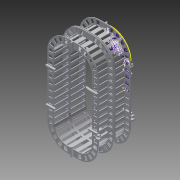
# Autodesk Inventor part: coil_former_hv_new
Saved by Autodesk Inventor 2014 SP1 (Build 180222100, 222)
## iProperties
Created: 2016-09-07
Part Number: coil_former_hv_new
Material: ABS Plastic
Document SubType Name: Modeling
Designer: tguillod
Density: 1.06 g/cm^3
Appearance: Smooth - White
Author: tguillod
Autodesk Inventor part; units mm, degrees
ref_plane "YZ Plane" through (0, 0, 0) normal (1, 0, 0) x (0, 1, 0)
ref_plane "XZ Plane" through (0, 0, 0) normal (0, 1, 0) x (-1, 0, 0)
ref_plane "XY Plane" through (0, 0, 0) normal (0, 0, 1) x (1, 0, 0)
sketch "Sketch1" plane through (0, 0, 0) normal (0, 0, 1) x (1, 0, 0)
  line L0 (0, 0) -> (10, 0)
  line L1 (10, 0) -> (10, 1)
  line L2 (10, 1) -> (1, 1)
  line L3 (1, 1) -> (1, 24.25)
  line L4 (1, 24.25) -> (10, 24.25)
  line L5 (10, 24.25) -> (10, 25.25)
  line L6 (10, 25.25) -> (1, 25.25)
  line L7 (1, 25.25) -> (1, 26.25)
  line L8 (1, 26.25) -> (10, 26.25)
  line L9 (10, 26.25) -> (10, 27.25)
  line L10 (10, 27.25) -> (1, 27.25)
  line L11 (1, 27.25) -> (1, 50.5)
  line L12 (1, 50.5) -> (10, 50.5)
  line L13 (10, 50.5) -> (10, 51.5)
  line L14 (10, 51.5) -> (0, 51.5)
  line L15 (0, 51.5) -> (0, 0)
  dimension "d0" = 10
  dimension "d1" = 9
  dimension "d2" = 1
  dimension "d3" = 1
  dimension "d4" = 1
  dimension "d5" = 1
  dimension "d6" = 1
  dimension "d7" = 51.5
  dimension "d8" = 23.25
  dimension "d9" = 23.25
  dimension "d10" = 1
  constraints: 32 end point, 11 parallel, 7 collinear, 1 horizontal, 1 perpendicular
  measures "d0" distance of L13.end L14.end
  measures "d1" distance of L9.end L10.end
  measures "d2" distance between parallel lines of L8 L6
  measures "d3" distance of L8.end L9.end
  measures "d4" distance of L12.end L13.end
  measures "d5" distance of L0.end L1.end
  measures "d6" distance of L4.end L5.end
  measures "d7" distance of L14.end L0.start
  measures "d8" distance between parallel lines of L2 L4
  measures "d9" distance between parallel lines of L12 L10
  measures "d10" distance between parallel lines of L15 L3
sketch "Sketch2" plane through (0, 0, 0) normal (0, 1, 0) x (-1, 0, 0)
  line L0 (0, 0) -> (0, 46.75)
  line L1 (22, 68.75) -> (30.5, 68.75)
  arc A0 (22, 68.75) -> (0, 46.75) centre (22, 46.75) ccw
  point P0 (0, 68.75)
  dimension "d11" = 68.75
  dimension "d12" = 30.5
  dimension "d13" = 22
  constraints: 4 end point, 2 point on circle, 2 point on line, 2 tangent, 1 centre point, 1 perpendicular, 1 vertical
  measures "d11" distance of L0.start point (0, 68.75)
  measures "d12" distance of point (0, 68.75) L1.end
  measures "d13" radius of A0
sweep "Sweep1" add profiles "Sketch1" path "Sketch2"
sketch "Sketch3" plane through (0, 51.5, 0) normal (0, 1, 0) x (1, 0, 0)
  line L0 (10, 0) -> (0, 0) projected
  line L1 (0, 0) -> (0, -46.75) projected
  line L2 (-22, -68.75) -> (-30.5, -68.75) projected
  line L3 (10, 0) -> (10, -46.75) projected
  line L4 (10, -28) -> (-4, -28)
  line L5 (-4, -28) -> (-4, -26)
  line L6 (-4, -26) -> (10, -26)
  line L7 (10, -26) -> (10, -28)
  line L8 (-30.5, -78.75) -> (-29.5, -78.75)
  line L9 (-29.5, -78.75) -> (-29.5, -64.75)
  line L10 (-29.5, -64.75) -> (-30.5, -64.75)
  line L11 (-30.5, -64.75) -> (-30.5, -78.75)
  dimension "d15" = 4
  dimension "d17" = 2
  dimension "d18" = 26
  dimension "d19" = 4
  dimension "d20" = 1
  constraints: 16 end point, 4 parallel, 2 horizontal, 2 perpendicular, 1 point on line
  measures "d15" distance between parallel lines of L5 L1
  measures "d17" distance between parallel lines of L4 L6
  measures "d18" distance between parallel lines of L6 L0
  measures "d19" distance between parallel lines of L10 L2
  measures "d20" distance of L9.end L10.end
extrude "Extrusion1" add sketch "Sketch3" along normal blind 3 contours L3 L4 L1 L6 | L1 L4 L5 L6 | L9 L8 L11 L2 | L2 L11 L10 L9
sketch "Sketch4" plane through (0, 0, 0) normal (0, -1, 0) x (1, 0, 0)
  line L0 (0, 0) -> (10, 0) projected
  line L1 (10, 0) -> (10, 46.75) projected
  line L2 (-22, 68.75) -> (-30.5, 68.75) projected
  line L3 (0, 0) -> (0, 46.75) projected
  line L4 (-30.5, 78.75) -> (-29.5, 78.75)
  line L5 (-29.5, 78.75) -> (-29.5, 64.75)
  line L6 (-29.5, 64.75) -> (-30.5, 64.75)
  line L7 (-30.5, 64.75) -> (-30.5, 78.75)
  line L8 (10, 28) -> (-4, 28)
  line L9 (-4, 28) -> (-4, 26)
  line L10 (-4, 26) -> (10, 26)
  line L11 (10, 26) -> (10, 28)
  dimension "d23" = 26
  dimension "d24" = 2
  dimension "d25" = 1
  dimension "d26" = 4
  dimension "d27" = 4
  constraints: 16 end point, 4 parallel, 2 horizontal, 2 perpendicular, 1 point on line
  measures "d23" distance between parallel lines of L0 L10
  measures "d24" distance of L8.end L9.end
  measures "d25" distance of L5.end L6.end
  measures "d26" distance between parallel lines of L2 L6
  measures "d27" distance between parallel lines of L3 L9
extrude "Extrusion2" add sketch "Sketch4" along normal blind 3 contours L10 L9 L8 L3 | L3 L8 L1 L10 | L5 L6 L7 L2 | L2 L7 L4 L5
sketch "Sketch19" plane through (0, 51.5, 28) normal (0, 1, 0) x (1, 0, 0)
  line L0 (0, 0) -> (0, -18.75) projected
  line L1 (-22, -40.75) -> (-29.5, -40.75) projected
  line L2 (-29.5, -40.75) -> (-29.5, -50.75) projected
  arc A0 (-22, -50.75) -> (10, -18.75) centre (-22, -18.75) ccw projected
  arc A1 (-22, -48.75) -> (-16.7906, -48.2942) centre (-22, -18.75) ccw
  line L3 (-22, -18.75) -> (-22, -48.75)
  line L4 (-22, -18.75) -> (-16.7906, -48.2942)
  arc A2 (-16.7906, -48.2942) -> (-11.7394, -46.9408) centre (-22, -18.75) ccw
  line L5 (-22, -18.75) -> (-11.7394, -46.9408)
  line L6 (-22, -18.75) -> (-16.7906, -48.2942)
  arc A3 (-11.7394, -46.9408) -> (-7, -44.7308) centre (-22, -18.75) ccw
  line L7 (-22, -18.75) -> (-7, -44.7308)
  line L8 (-22, -18.75) -> (-11.7394, -46.9408)
  arc A4 (-7, -44.7308) -> (-2.7164, -41.7313) centre (-22, -18.75) ccw
  line L9 (-22, -18.75) -> (-2.7164, -41.7313)
  line L10 (-22, -18.75) -> (-7, -44.7308)
  arc A5 (-2.7164, -41.7313) -> (0.9813, -38.0336) centre (-22, -18.75) ccw
  line L11 (-22, -18.75) -> (0.9813, -38.0336)
  line L12 (-22, -18.75) -> (-2.7164, -41.7313)
  arc A6 (0.9813, -38.0336) -> (3.9808, -33.75) centre (-22, -18.75) ccw
  line L13 (-22, -18.75) -> (3.9808, -33.75)
  line L14 (-22, -18.75) -> (0.9813, -38.0336)
  arc A7 (3.9808, -33.75) -> (6.1908, -29.0106) centre (-22, -18.75) ccw
  line L15 (-22, -18.75) -> (6.1908, -29.0106)
  line L16 (-22, -18.75) -> (3.9808, -33.75)
  arc A8 (6.1908, -29.0106) -> (7.5442, -23.9594) centre (-22, -18.75) ccw
  line L17 (-22, -18.75) -> (7.5442, -23.9594)
  line L18 (-22, -18.75) -> (6.1908, -29.0106)
  arc A9 (7.5442, -23.9594) -> (8, -18.75) centre (-22, -18.75) ccw
  line L19 (-22, -18.75) -> (8, -18.75)
  line L20 (-22, -18.75) -> (7.5442, -23.9594)
  line L21 (-28, -40.75) -> (-30.5, -40.75)
  line L22 (-30.5, -40.75) -> (-30.5, -42.75)
  line L23 (-30.5, -42.75) -> (-28, -42.75)
  line L24 (-28, -42.75) -> (-28, -40.75)
  line L25 (0, -14.75) -> (8, -14.75)
  line L26 (8, -14.75) -> (8, -10.25)
  line L27 (8, -10.25) -> (0, -10.25)
  line L28 (0, -10.25) -> (0, -14.75)
  line L29 (0, -5.75) -> (8, -5.75)
  line L30 (8, -5.75) -> (8, -1.25)
  line L31 (8, -1.25) -> (0, -1.25)
  line L32 (0, -1.25) -> (0, -5.75)
  line L33 (0, 3.25) -> (8, 3.25)
  line L34 (8, 3.25) -> (8, 7.75)
  line L35 (8, 7.75) -> (0, 7.75)
  line L36 (0, 7.75) -> (0, 3.25)
  line L37 (0, 12.25) -> (8, 12.25)
  line L38 (8, 12.25) -> (8, 16.75)
  line L39 (8, 16.75) -> (0, 16.75)
  line L40 (0, 16.75) -> (0, 12.25)
  line L41 (0, 21.25) -> (8, 21.25)
  line L42 (8, 21.25) -> (8, 25.75)
  line L43 (8, 25.75) -> (0, 25.75)
  line L44 (0, 25.75) -> (0, 21.25)
  line L45 (0, 2) -> (10, 2) projected
  line L46 (8, 25.75) -> (2, 25.75)
  line L47 (2, 25.75) -> (2, 21.25)
  line L48 (2, 21.25) -> (8, 21.25)
  line L49 (8, 21.25) -> (8, 25.75)
  line L50 (8, 16.75) -> (2, 16.75)
  line L51 (2, 16.75) -> (2, 12.25)
  line L52 (2, 12.25) -> (8, 12.25)
  line L53 (8, 12.25) -> (8, 16.75)
  line L54 (8, 7.75) -> (2, 7.75)
  line L55 (2, 7.75) -> (2, 3.25)
  line L56 (2, 3.25) -> (8, 3.25)
  line L57 (8, 3.25) -> (8, 7.75)
  line L58 (8, -1.25) -> (2, -1.25)
  line L59 (2, 2) -> (8, 2)
  line L60 (8, -10.25) -> (2, -10.25)
  line L61 (2, -10.25) -> (2, -14.75)
  line L62 (2, -14.75) -> (8, -14.75)
  line L63 (8, -14.75) -> (8, -10.25)
  line L64 (0, 28) -> (0, 2) projected
  arc A10 (-22, -42.75) -> (-17.8324, -42.3854) centre (-22, -18.75) ccw
  arc A11 (-13.7915, -41.3026) -> (-10, -39.5346) centre (-22, -18.75) ccw
  arc A12 (-6.5731, -37.1351) -> (-3.6149, -34.1769) centre (-22, -18.75) ccw
  arc A13 (-1.2154, -30.75) -> (0.5526, -26.9585) centre (-22, -18.75) ccw
  arc A14 (1.6354, -22.9176) -> (2, -18.75) centre (-22, -18.75) ccw
  line L65 (-22, -42.75) -> (-22, -48.75)
  line L66 (-17.8324, -42.3854) -> (-16.7906, -48.2942)
  line L67 (2, -18.75) -> (8, -18.75)
  line L68 (1.6354, -22.9176) -> (7.5442, -23.9594)
  line L69 (0.5526, -26.9585) -> (6.1908, -29.0106)
  line L70 (-1.2154, -30.75) -> (3.9808, -33.75)
  line L71 (-3.6149, -34.1769) -> (0.9813, -38.0336)
  line L72 (-2.7164, -41.7313) -> (-6.5731, -37.1351)
  line L73 (-7, -44.7308) -> (-10, -39.5346)
  line L74 (-13.7915, -41.3026) -> (-11.7394, -46.9408)
  line L75 (8, -1.25) -> (2, -1.25)
  line L76 (2, -1.25) -> (2, -5.75)
  line L77 (2, -5.75) -> (8, -5.75)
  line L78 (8, -5.75) -> (8, -1.25)
  dimension "d112" = 10
  dimension "d113" = 10
  dimension "d114" = 10
  dimension "d115" = 10
  dimension "d116" = 10
  dimension "d117" = 10
  dimension "d118" = 10
  dimension "d119" = 10
  dimension "d120" = 10
  dimension "d121" = 30
  dimension "d122" = 1
  dimension "d123" = 1.5
  dimension "d124" = 2
  dimension "d125" = 8
  dimension "d126" = 4.5
  dimension "d127" = 4
  dimension "d130" = 9
  dimension "d143" = 2
  dimension "d144" = 24
  constraints: 148 end point, 28 point on circle, 15 parallel, 14 centre point, 14 coincident, 14 collinear, 13 point on line, 8 horizontal, 8 perpendicular, 4 concentric, 1 vertical, 32 other
  measures "d112" angle of L3 L4
  measures "d113" angle of L6 L5
  measures "d114" angle of L8 L7
  measures "d115" angle of L10 L9
  measures "d116" angle of L12 L11
  measures "d117" angle of L14 L13
  measures "d118" angle of L16 L15
  measures "d119" angle of L18 L17
  measures "d120" angle of L20 L19
  measures "d121" radius of A1
  measures "d122" distance between parallel lines of L22 L2
  measures "d123" distance between parallel lines of L24 L2
  measures "d124" distance of L23.end L21.start
  measures "d125" distance of L25.start L25.end
  measures "d126" distance of L25.end L26.end
  measures "d127" distance from line of L0.end L25
  measures "d130" distance of L25.start L29.start
  measures "d143" distance between parallel lines of L64 L47
  measures "d144" radius of A10
extrude "Extrusion13" cut sketch "Sketch19" against normal up to surface (23.25 mm away) from surface at -1 contours L31 L76 L29 L0 | L31 L30 L29 L76 | L27 L61 L25 L0 | L27 L26 L25 L61 | L24 L23 L2 L1 | L2 L23 L22 L21 | L3 A10 L4 A1 | L3 L4 A10 | L5 A11 L7 A3 | L7 A11 L5 | L11 A12 L9 | L15 A13 L13 | L19 A14 L17 | A12 L11 A5 L9 | A13 L15 A7 L13 | A14 L19 A9 L17 | L36 L35 L55 L33 | L55 L35 L34 L33 | L40 L39 L51 L37 | L51 L39 L38 L37 | L44 L43 L47 L41 | L47 L43 L42 L41
extrude "Extrusion14" cut sketch "Sketch19" against normal up to surface (23.25 mm away) from surface at -27.25 contours L31 L76 L29 L0 | L31 L30 L29 L76 | L27 L61 L25 L0 | L27 L26 L25 L61 | L24 L23 L2 L1 | L2 L23 L22 L21 | L3 A10 L4 A1 | L3 L4 A10 | L5 A11 L7 A3 | L7 A11 L5 | L11 A12 L9 | L15 A13 L13 | L19 A14 L17 | A12 L11 A5 L9 | A13 L15 A7 L13 | A14 L19 A9 L17 | L36 L35 L55 L33 | L55 L35 L34 L33 | L40 L39 L51 L37 | L51 L39 L38 L37 | L44 L43 L47 L41 | L47 L43 L42 L41
extrude "Extrusion15" cut sketch "Sketch19" against normal through all contours L31 L30 L29 L76 | L27 L26 L25 L61 | L55 L35 L34 L33 | L51 L39 L38 L37 | L47 L43 L42 L41
extrude "Extrusion16" cut sketch "Sketch19" against normal through all contours L3 A10 L4 A1 | L5 A11 L7 A3 | A12 L11 A5 L9 | A13 L15 A7 L13 | A14 L19 A9 L17
mirror "Mirror1" about plane through (-30.5, 25.75, 71.4873) normal (-1, 0, 0)
mirror "Mirror2" about plane through (2.7373, 25.75, 0) normal (0, 0, -1)
sketch "Sketch21" plane through (10, 51.5, 26) normal (1, 0, 0) x (0, 0, -1)
  line L0 (72.75, -1) -> (-20.75, -1) projected
  line L1 (72.75, -1) -> (72.75, 0) projected
  line L2 (54, 0) -> (54, 3) projected
  line L3 (54, 3) -> (52, 3) projected
  line L4 (72.75, -50.5) -> (-20.75, -50.5) projected
  line L5 (-20.75, -51.5) -> (-20.75, -50.5) projected
  line L6 (-2, -51.5) -> (-20.75, -51.5) projected
  line L7 (-2, -51.5) -> (-2, -54.5) projected
  line L8 (0, -54.5) -> (-2, -54.5) projected
  line L9 (0, -51.5) -> (0, -54.5) projected
  line L10 (52, -51.5) -> (0, -51.5) projected
  line L11 (52, -51.5) -> (52, -54.5) projected
  line L12 (52, -54.5) -> (54, -54.5) projected
  line L13 (54, -51.5) -> (54, -54.5) projected
  line L14 (54, -51.5) -> (72.75, -51.5) projected
  line L15 (72.75, -51.5) -> (72.75, -50.5) projected
  line L16 (61, -1) -> (59, -1)
  line L17 (59, -1) -> (59, 3)
  line L18 (59, 3) -> (61, 3)
  line L19 (61, 3) -> (61, -1)
  line L20 (54, -1) -> (56, -1)
  line L21 (56, -1) -> (56, 3)
  line L22 (56, 3) -> (54, 3)
  line L23 (54, 3) -> (54, -1)
  line L24 (56, -50.5) -> (54, -50.5)
  line L25 (54, -50.5) -> (54, -54.5)
  line L26 (54, -54.5) -> (56, -54.5)
  line L27 (56, -54.5) -> (56, -50.5)
  line L28 (61, -50.5) -> (59, -50.5)
  line L29 (59, -50.5) -> (59, -54.5)
  line L30 (59, -54.5) -> (61, -54.5)
  line L31 (61, -54.5) -> (61, -50.5)
  point P0 (26, -51.5)
  dimension "d155" = 11.75
  dimension "d156" = 3
  dimension "d157" = 2
  dimension "d158" = 2
  dimension "d163" = 2
  constraints: 32 end point, 9 parallel, 7 collinear, 4 horizontal, 4 perpendicular, 4 point on line
  measures "d155" distance between parallel lines of L19 L1
  measures "d156" distance between parallel lines of L17 L21
  measures "d157" distance of L17.end L18.end
  measures "d158" distance of L29.end L30.end
  measures "d163" distance of L21.end L22.end
extrude "Extrusion18" add sketch "Sketch21" along normal blind 3 and the other way blind 2 contours L0 L17 L18 L19 | L0 L23 L2 L22 L21 | L31 L14 L29 L4 | L31 L30 L29 L14 | L27 L14 L25 L4 | L27 L26 L13 L14
sketch "Sketch22" plane through (-39, 27.25, 78.75) normal (0, 1, 0) x (1, 0, 0)
  line L0 (40, 112.5) -> (41, 112.5)
  line L1 (41, 112.5) -> (41, 108)
  line L2 (41, 108) -> (40, 108)
  line L3 (40, 108) -> (40, 112.5)
  point P0 (39, 78.75)
  constraints: 8 end point, 2 parallel, 1 horizontal, 1 perpendicular
extrude "Extrusion19" cut sketch "Sketch22" against normal blind 10
body "Solid1"
